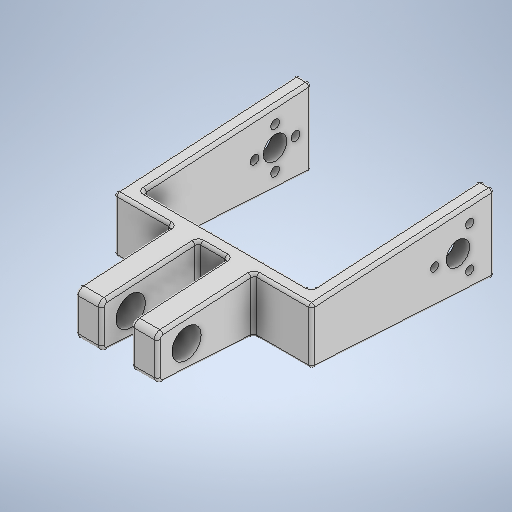
# Autodesk Inventor part: Braço do motor II
Saved by Autodesk Inventor 2025.3 (Build 293356000, 356)
## iProperties
Created: 2025-03-23
Part Number: Braço do motor II
Material: Generic
Document SubType Name: Modeling
Designer: erikg
Density: 1 g/cm^3
Appearance: Default
Author: erikg
Autodesk Inventor part; units mm, degrees
ref_plane "YZ Plane" through (0, 0, 0) normal (1, 0, 0) x (0, 1, 0)
ref_plane "XZ Plane" through (0, 0, 0) normal (0, 1, 0) x (-1, 0, 0)
ref_plane "XY Plane" through (0, 0, 0) normal (0, 0, 1) x (1, 0, 0)
sketch "Sketch1" plane through (0, 0, 0) normal (1, 0, 0) x (0, 1, 0)
  circle A0 centre (0, -53.3311) radius 12.5
  line L0 (-7.5, 29.6689) -> (7.5, 29.6689)
  line L1 (7.5, 29.6689) -> (12.4772, -52.5761)
  line L2 (-12.4772, -52.5761) -> (-7.5, 29.6689)
  line L3 (12.4772, -52.5761) -> (13.2793, -65.8311)
  line L4 (-12.4772, -52.5761) -> (-13.2793, -65.8311)
  line L5 (-13.2793, -65.8311) -> (13.2793, -65.8311)
  point P0 (0, 0)
  point P1 (0, 29.6689)
  point P2 (-12.4096, -51.8306)
  point P3 (12.4096, -51.8306)
  point P4 (0, -65.8311)
  point P5 (-12.5, -53.3311)
  point P6 (0.1991, -65.8295)
  dimension "d0" = 25
  dimension "d1" = 15
  dimension "d2" = 83
  constraints: 12 end point, 3 point on circle, 3 point on line, 3 tangent, 2 horizontal, 2 vertical alignment, 1 centre point, 1 midpoint
  measures "d0" diameter of A0
  measures "d1" distance of L0.start L0.end
  measures "d2" distance from line of L0 A0.centre
extrude "Extrusion1" add sketch "Sketch1" along normal mid plane 67.5
sketch "Sketch3" plane through (33.75, 0, 0) normal (1, 0, 0) x (0, 0, -1)
  arc A0 (65.8295, -0.1991) -> (65.8295, 0.1991) centre (53.3311, 0) ccw projected
  point P0 (0, 0)
  point P1 (51.8306, -12.4096)
  point P2 (51.8306, 12.4096)
  point P3 (53.3311, -12.5)
  point P4 (52.5761, 12.4772)
  constraints: 1 coincident
hole "Hole1" at (33.75, 0, -53.3311) direction (-1, 0, 0) diameter 8 end through all
sketch "Sketch4" plane through (0, 0, 0) normal (0, 1, 0) x (-1, 0, 0)
  line L0 (28.75, -8.3311) -> (-28.75, -8.3311)
  line L1 (-28.75, -8.3311) -> (-28.75, -79.7826)
  line L2 (-28.75, -79.7826) -> (28.75, -79.7826)
  line L3 (28.75, -79.7826) -> (28.75, -8.3311)
  line L4 (33.75, 29.6689) -> (-33.75, 29.6689) projected
  line L5 (33.75, -65.8311) -> (33.75, 29.6689) projected
  line L6 (-33.75, 29.6689) -> (-33.75, -65.8311) projected
  line L7 (33.75, 29.6689) -> (14, 29.6689)
  line L8 (14, 29.6689) -> (14, -3.3311)
  line L9 (14, -3.3311) -> (33.75, -3.3311)
  line L10 (33.75, -3.3311) -> (33.75, 29.6689)
  line L11 (-33.75, 29.6689) -> (-14, 29.6689)
  line L12 (-14, 29.6689) -> (-14, -3.3311)
  line L13 (-14, -3.3311) -> (-33.75, -3.3311)
  line L14 (-33.75, -3.3311) -> (-33.75, 29.6689)
  line L15 (5.1, 29.6689) -> (-5.1, 29.6689)
  line L16 (-5.1, 29.6689) -> (-5.1, -3.3311)
  line L17 (-5.1, -3.3311) -> (5.1, -3.3311)
  line L18 (5.1, -3.3311) -> (5.1, 29.6689)
  point P0 (0, 0)
  point P1 (33.75, -51.8306)
  point P2 (-33.75, -51.8306)
  point P3 (0, -3.3311)
  dimension "d13" = 38
  dimension "d14" = 5
  dimension "d15" = 5
  dimension "d18" = 19.75
  dimension "d19" = 33
  dimension "d20" = 10.2
  constraints: 32 end point, 8 parallel, 4 horizontal, 4 perpendicular, 2 equal length, 2 point on line, 1 midpoint, 1 vertical alignment
  measures "d13" distance between parallel lines of L4 L0
  measures "d14" distance between parallel lines of L5 L3
  measures "d15" distance between parallel lines of L6 L1
  measures "d18" distance of L8.end L9.end
  measures "d19" distance of L7.end L8.end
  measures "d20" distance of L16.end L17.end
extrude "Extrusion2" cut sketch "Sketch4" along normal through all both and the other way through all
sketch "Sketch5" plane through (14, -9.497, -3.3311) normal (1, 0, 0) x (0, 0, -1)
  line L0 (-33, 1.997) -> (-33, 16.997) projected
  point P0 (-3.3311, 9.497)
  point P1 (-23, 9.497)
  point P2 (-33, 16.988)
  dimension "d21" = 10
  constraints: 1 horizontal alignment
  measures "d21" distance from line of L0 point (-23, 9.497)
hole "Hole2" at (14, 0, 19.6689) direction (-1, 0, 0) diameter 10 end through all
fillet "Fillet1" radius 2 4 edges at (9.55, 7.5, 29.6689) (9.55, -7.5, 29.6689) (-9.55, -7.5, 29.6689) (-9.55, 7.5, 29.6689)
fillet "Fillet2" radius 1 22 edges at (14, 0, -3.3311) (-14, 0, -3.3311) (-5.1, 0, -3.3311) (5.1, 0, -3.3311) (-28.75, 0, -8.3311) (28.75, 0, -8.3311) (0, 9.7996, -8.3311) (0, -9.7996, -8.3311) (-28.75, 11.5395, -37.0811) (28.75, 11.5395, -37.0811) (28.75, -11.5395, -37.0811) (-28.75, -11.5395, -37.0811) (23.875, -9.497, -3.3311) (33.75, -11.3882, -34.5811) (-23.875, -9.497, -3.3311) (-33.75, -11.3882, -34.5811) (23.875, 9.497, -3.3311) (33.75, 11.3882, -34.5811) (-23.875, 9.497, -3.3311) (-33.75, 11.3882, -34.5811) (-33.75, 0, -3.3311) (33.75, 0, -3.3311)
fillet "Fillet3" radius 1 31 edges at (-23.875, -9.5539, -4.2707) (-13.5733, -9.5177, -3.6717) (-4.8071, 9.4793, -3.0382) (4.8071, 9.4793, -3.0382) (-32.75, 11.4166, -35.0509) (-23.875, 9.5539, -4.2707) (-13.5733, 9.5177, -3.6717) (-13, 8.5233, 12.7595) (-29.1492, 9.7701, -7.8431) (0, 9.7355, -7.2707) (29.1492, 9.7701, -7.8431) (23.875, 9.5539, -4.2707) (13, 8.5233, 12.7595) (13.5733, 9.5177, -3.6717) (32.75, -11.4166, -35.0509) (23.875, -9.5539, -4.2707) (13.5733, -9.5177, -3.6717) (4.8071, -9.4793, -3.0382) (0, -9.497, -3.3311) (-4.8071, -9.4793, -3.0382) (-5.1, -8.5251, 12.7293) (-5.1, -6.9882, 29.1252) (-5.1, 0, 29.6689) (-5.1, 6.9882, 29.1252) (-5.1, 8.5251, 12.7293) (0, 9.497, -3.3311) (5.1, 8.5251, 12.7293) (5.1, 6.9882, 29.1252) (5.1, 0, 29.6689) (5.1, -6.9882, 29.1252) (5.1, -8.5251, 12.7293)
sketch "Sketch6" plane through (-33.75, 0, 0) normal (-1, 0, 0) x (0, 0, 1)
  circle A0 centre (-53.3311, 0) radius 4 projected
  circle A1 centre (-53.3311, 0) radius 1.4138
  point P0 (0, 0)
  point P1 (-53.3311, -7)
  point P2 (-46.3311, 0)
  point P3 (-53.3311, 7)
  point P4 (-60.3311, 0)
  dimension "d32" = 7
  dimension "d35" = 360
  constraints: 1 centre point, 1 coincident, 5 other
  measures "d32" vertical distance of point (0, 0) point (-53.331, -7)
hole "Hole3" at (-33.75, -7, -53.3311) at (-33.75, 0, -46.3311) at (-33.75, 7, -53.3311) at (-33.75, 0, -60.3311) direction (1, 0, 0) diameter 3 depth 5
sketch "Sketch7" plane through (33.75, 0, 0) normal (1, 0, 0) x (0, 0, -1)
  circle A0 centre (53.3311, 0) radius 4 projected
  point P0 (0, 0)
  point P1 (45.3311, 0)
  point P2 (57.3311, -6.9282)
  point P3 (57.3311, 6.9282)
  dimension "d44" = 8
  dimension "d47" = 360
  constraints: 4 other
  measures "d44" distance of A0.centre point (45.331, 0)
hole "Hole4" at (33.75, 0, -45.3311) at (33.75, -6.9282, -57.3311) at (33.75, 6.9282, -57.3311) direction (-1, 0, 0) diameter 2.8 depth 5
fillet "Fillet4" radius 1 14 edges at (29.0429, -12.9859, -65.8311) (29.0429, 12.9859, -65.8311) (-31.25, -13.2793, -65.8311) (31.25, -13.2793, -65.8311) (33.4571, -12.9859, -65.8311) (33.75, 0, -65.8311) (-31.25, 13.2793, -65.8311) (31.25, 13.2793, -65.8311) (28.75, 0, -65.8311) (-29.0429, -12.9859, -65.8311) (-29.0429, 12.9859, -65.8311) (-33.4571, -12.9859, -65.8311) (-33.75, 0, -65.8311) (-28.75, 0, -65.8311)
body "Solid1"
